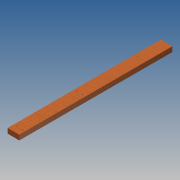
# Autodesk Inventor part: 2p2psh2
Saved by Autodesk Inventor 2014 SP1 (Build 180222100, 222)
## iProperties
Company: HERA Project
Created: 2013-09-03
Part Number: 2p2psh2
Material: Wood (Cherry)
Document SubType Name: Modeling
Designer: David DeBoer
Mass: 2056.37 g
Surface Area: 3183.04 cm^2
Volume: 4112.74 cm^3
Density: 0.5 g/cm^3
Description: pole stand support horizontal 2
Appearance: Cherry - Natural Low Gloss
Author: David DeBoer
Autodesk Inventor part; units mm, degrees
ref_plane "YZ Plane" through (0, 0, 0) normal (1, 0, 0) x (0, 1, 0)
ref_plane "XZ Plane" through (0, 0, 0) normal (0, 1, 0) x (-1, 0, 0)
ref_plane "XY Plane" through (0, 0, 0) normal (0, 0, 1) x (1, 0, 0)
sketch "Sketch1" plane through (0, 0, 0) normal (1, 0, 0) x (0, 1, 0)
  line L0 (0, 0) -> (38.1, 0)
  line L1 (38.1, 0) -> (38.1, -1168.4)
  line L2 (38.1, -1168.4) -> (0, -1168.4) construction
  line L3 (0, -1168.4) -> (0, 0)
  line L4 (0, -1168.4) -> (38.1, -1168.4)
  line L5 (0, -1168.4) -> (104.052, -1168.4) construction
  dimension "d0" = 38.1
  dimension "d1" = 1168.4
  dimension "d3" = 90
  constraints: 12 end point, 2 horizontal, 2 parallel, 1 perpendicular
  measures "d0" distance of L0.start L0.end
  measures "d1" distance of L2.end L0.start
  measures "d3" angle of L4 L3
extrude "Extrusion1" add sketch "Sketch1" along normal blind 88.9
sketch "Sketch4" plane through (0, 38.1, 0) normal (0, 1, 0) x (1, 0, 0)
  line L0 (0, 0) -> (0, 1168.4) projected
  line L1 (0, 0) -> (88.9, 0) projected
  circle A0 centre (22.225, 49.4696) radius 8.5666
  circle A1 centre (66.675, 49.4696) radius 8.5666
  circle A2 centre (22.225, 506.6696) radius 8.5666
  circle A3 centre (66.675, 506.6696) radius 8.5666
  dimension "d46" = 22.225
  dimension "d49" = 44.45
  dimension "d52" = 457.2
  constraints: 4 centre point, 1 horizontal, 1 vertical, 6 other
  measures "d46" distance from line of L0 A0.centre
  measures "d49" distance of A0.centre A1.centre
  measures "d52" distance of A0.centre A2.centre
hole "Hole3" at (22.225, 38.1, -49.4696) at (66.675, 38.1, -49.4696) at (22.225, 38.1, -506.6696) at (66.675, 38.1, -506.6696) direction (0, -1, 0) diameter 6.7564 end through all clearance for "Flat Head Machine Screw (82)" size "1/4" standard "Ansi Unified Screw Threads"
equation "\"d46\" = 0.25 * d4"
equation "\"d49\" = 0.5 * d4"
equation "\"d4\" = 88.9"
body "Solid1"
